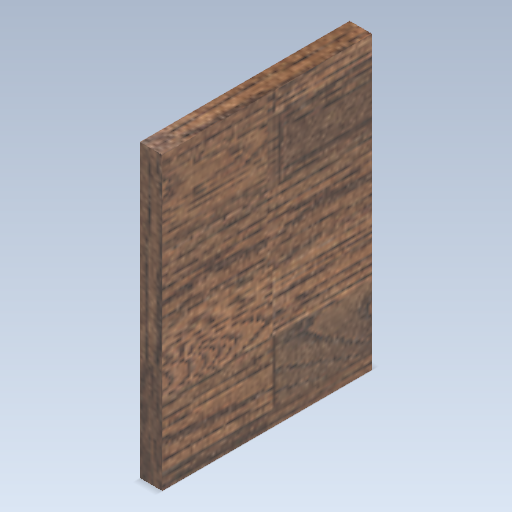
# Autodesk Inventor part: Battery Box Cover
Saved by Autodesk Inventor 2020 (Build 240168000, 168)
## iProperties
Created: 2020-08-16
Part Number: Battery Box Cover
Material: Generic
Document SubType Name: Modeling
Designer: Abbas
Density: 1 g/cm^3
Appearance: Default
Author: Abbas
Autodesk Inventor part; units mm, degrees
ref_plane "YZ Plane" through (0, 0, 0) normal (1, 0, 0) x (0, 1, 0)
ref_plane "XZ Plane" through (0, 0, 0) normal (0, 1, 0) x (-1, 0, 0)
ref_plane "XY Plane" through (0, 0, 0) normal (0, 0, 1) x (1, 0, 0)
sketch "Sketch1" plane through (0, 0, 0) normal (1, 0, 0) x (0, 1, 0)
  line L0 (-130, 92.222) -> (-130, -95)
  line L1 (-130, -95) -> (130, -95)
  line L2 (130, -95) -> (130, 92.222)
  line L3 (130, 92.222) -> (-130, 92.222)
  point P0 (0, 0)
  dimension "d0" = 260
  constraints: 8 end point, 1 parallel
  measures "d0" distance of L1.end L0.end
extrude "Extrusion1" add sketch "Sketch1" along normal blind 20
sketch "Sketch2" plane through (0, -130, -95) normal (0, 0, -1) x (-1, 0, 0)
  circle A0 centre (-12.5, 244.99) radius 1.875
  circle A1 centre (-12.5, 219.19) radius 1.875
  circle A2 centre (-12.5, 193.39) radius 1.875
  line L0 (0, 260) -> (-20, 260) projected
  line L1 (0, 0) -> (0, 260) projected
  point P0 (0, 130)
  dimension "d4" = 3.75
  dimension "d5" = 3.75
  dimension "d6" = 3.75
  dimension "d7" = 15.01
  dimension "d8" = 25.8
  dimension "d9" = 25.8
  dimension "d10" = 12.5
  constraints: 3 centre point
  measures "d4" diameter of A0
  measures "d5" diameter of A1
  measures "d6" diameter of A2
  measures "d7" distance from line of L0 A0.centre
  measures "d8" distance of A0.centre A1.centre
  measures "d9" distance of A2.centre A1.centre
  measures "d10" distance from line of L1 A0.centre
extrude "Extrusion2" cut sketch "Sketch2" against normal blind 10
body "Solid1"
